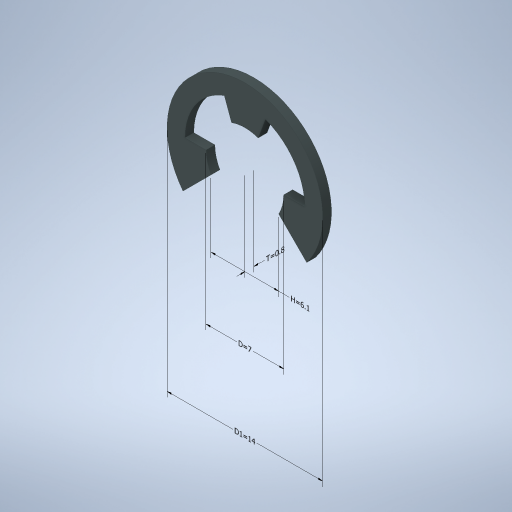
# Autodesk Inventor part: METW-7
Saved by Autodesk Inventor 2023 (Build 270158000, 158)
## iProperties
Category: PARTsolutions
Company: TOHATSU
Created: 2023-07-21
Part Number: METW-7
Material: Generic
Catalog Web Link: www.cadenas.de
Description: METW．METWS．CAP-METW．CAP-METWS-E-type Buckle
Vendor: TOHATSU
Document SubType Name: Modeling
Designer: psAdmin
Manufacturer: TOHATSU
Mass: 0.372348 g
Surface Area: 1.70625 cm^2
Volume: 0.0474329 cm^3
Density: 7.85 g/cm^3
Appearance: PSOLRGB-76-89-91
PSOL_IDENT_0: {$CADENAS_DATA/23d-libs/tohatsu/machinery-components/locating-fixed-components/retaining-ring/metw.p
PSOL_IDENT_1: rj},176 {VTYP=3D},{NB=METW-7},{LINA=METW-7},{NN=METW．METWS．CAP-METW．CAP-METWS},{DATE=09.12.2022 05:3
PSOL_IDENT_2: 7:07},{GEOMDATE=09.12.2022 05:31:06},{VERSION=},{LINEID=930},{WBVAR=},{WBNUMERIC=}  {NB=METW-7},{LIN
PSOL_IDENT_3: A=METW-7},{KT=DUMMY},{PN=METW-7},{ROHS=YES},{TYPE=METW},{MA=彈簧鋼},{QU=7850},{PS=散裝},{COL=0.30,0.35,0.
PSOL_IDENT_4: 36,0.00},{NO=7.0},{D=7.0},{D1=14},{H=6.1},{T=0.8},{D3=1.6},{URL=https://www.tohatsu.com.tw},{WED=網站}
NB: METW-7
NN: METW．METWS．CAP-METW．CAP-METWS
NT: E-type Buckle
NBSYN: $PN.
LINA: METW-7
CATALOG: TOHATSU
PN: METW-7
ROHS: YES
TYPE: METW
MA: Spring Steel
PS: Bulk
NO: 7
D: 7
T: 0.8
WED: 網站
SUPPLIER: TOHATSU
ARTICLENO: METW-7
BOMINFO: METW-7
CREATOR: CADENAS GmbH
Title: METW-7
Author: Cadenas PARTsolutions
Comments: E-type Buckle
Autodesk Inventor part; units mm, degrees
ref_plane "YZ Plane" through (0, 0, 0) normal (1, 0, 0) x (0, 1, 0)
ref_plane "XZ Plane" through (0, 0, 0) normal (0, 1, 0) x (-1, 0, 0)
ref_plane "XY Plane" through (0, 0, 0) normal (0, 0, 1) x (1, 0, 0)
sketch "__1" plane through (0, 0, 0) normal (0, 0, 1) x (1, 0, 0)
  arc A0 (5.5712, -4.2381) -> (-5.5712, -4.2381) centre (0, 0) ccw
  line L0 (-5.5712, -4.2381) -> (-3.05, -1.7168)
  arc A1 (-3.5, 0) -> (-3.05, -1.7168) centre (0, 0) ccw
  line L1 (-3.5, 0) -> (-5.4, 0)
  arc A2 (-1.8469, 5.0743) -> (-5.4, 0) centre (0, 0) ccw
  line L2 (-1.8469, 5.0743) -> (-1.1971, 3.2889)
  arc A3 (1.1971, 3.2889) -> (-1.1971, 3.2889) centre (0, 0) ccw
  line L3 (1.1971, 3.2889) -> (1.8469, 5.0743)
  arc A4 (5.4, 0) -> (1.8469, 5.0743) centre (0, 0) ccw
  line L4 (5.4, 0) -> (3.5, 0)
  arc A5 (3.05, -1.7168) -> (3.5, 0) centre (0, 0) ccw
  line L5 (3.05, -1.7168) -> (5.5712, -4.2381)
  constraints: 12 end point, 12 point on circle, 6 centre point
extrude "Extrusion1" add sketch "__1" against normal blind 0.8
ref_plane "CA3_XY" through (0, 0, -0.4) normal (-1, 0, 0) x (0, 0, -1)
ref_plane "CA3_YZ" through (0, 0, -0.4) normal (0, 0, -1) x (0, -1, 0)
ref_plane "CA3_ZX" through (0, 0, -0.4) normal (0, -1, 0) x (-1, 0, 0)
body "Solid1"
